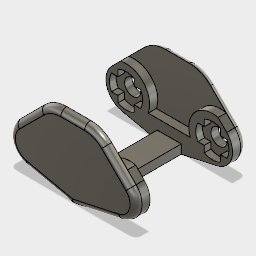
servo_bracket_shin (Autodesk Fusion 360 design; units mm, degrees)
Autodesk Fusion 360 part; units mm, degrees
sketch "スケッチ1" plane through (0, 0, 0) normal (0, 0, 1) x (1, 0, 0)
  line L0 (0, 0) -> (-4, 0)
  line L1 (0, 0) -> (4, 0)
  line L2 (-4, 0) -> (-15.8267, 2.557)
  line L3 (-4, 0) -> (8.1, 0) construction
  line L4 (4, 0) -> (15.8267, 2.557)
  line L5 (4, 0) -> (16.1, 0) construction
  line L6 (-15.8267, 2.557) -> (-14.4003, 9.1546)
  line L7 (15.8267, 2.557) -> (14.4003, 9.1546)
  circle A0 centre (14.4003, 9.1546) radius 6.75
  circle A1 centre (-14.4003, 9.1546) radius 6.75
  line L8 (14.4003, 9.1546) -> (15.8267, 2.557)
  line L9 (14.4003, 9.1546) -> (19.1733, 13.9276)
  line L10 (14.4003, 9.1546) -> (21.1503, 9.1546) construction
  line L11 (-14.4003, 9.1546) -> (-19.1733, 13.9276)
  line L12 (-14.4003, 9.1546) -> (-7.6503, 9.1546) construction
  line L13 (19.1733, 13.9276) -> (11.0592, 22.0416)
  line L14 (11.0592, 22.0416) -> (3.9881, 14.9705)
  line L15 (11.0592, 22.0416) -> (21.0592, 22.0416) construction
  line L16 (3.9881, 14.9705) -> (3.9881, 24.9705)
  arc A2 (11.0592, 22.0416) -> (3.9881, 24.9705) centre (3.9881, 14.9705) ccw
  line L17 (-19.1733, 13.9276) -> (-11.0592, 22.0416)
  line L18 (-11.0592, 22.0416) -> (-3.9881, 14.9705)
  line L19 (-3.9881, 14.9705) -> (-3.9881, 24.9705)
  line L20 (-3.9881, 24.9705) -> (3.9881, 24.9705)
  arc A3 (-3.9881, 24.9705) -> (-11.0592, 22.0416) centre (-3.9881, 14.9705) ccw
  circle A4 centre (-14.4003, 9.1546) radius 2.7
  circle A5 centre (14.4003, 9.1546) radius 2.7
  circle A6 centre (-14.4003, 9.1546) radius 2
  circle A7 centre (14.4003, 9.1546) radius 2
  circle A8 centre (-14.4003, 9.1546) radius 7.875
  circle A9 centre (14.4003, 9.1546) radius 7.875
  line L21 (0, 0) -> (0, 6.4) construction
  line L22 (0, 6.4) -> (-7.0228, 6.4)
  line L23 (0, 6.4) -> (7.0228, 6.4)
  line L24 (-4, 0) -> (4, 0)
  line L25 (4, 0) -> (4, 3)
  line L26 (4, 3) -> (-4, 3)
  line L27 (-4, 3) -> (-4, 0)
  dimension "d1" = 4
  dimension "d2" = 4
  dimension "d3" = 167.8
  dimension "d4" = 12.1
  dimension "d5" = 12.2
  dimension "d6" = 12.1
  dimension "d7" = 6.75
  dimension "d8" = 6.75
  dimension "d9" = 6.75
  dimension "d10" = 45
  dimension "d11" = 6.75
  dimension "d12" = 135
  dimension "d13" = 11.475
  dimension "d16" = 10
  dimension "d18" = 10
  dimension "d19" = 11.475
  dimension "d20" = 10
  dimension "d21" = 10
  dimension "d28" = 5.4
  dimension "d29" = 5.4
  dimension "d30" = 4
  dimension "d31" = 4
  dimension "d32" = 15.75
  dimension "d33" = 15.75
  dimension "d34" = 6.4
  dimension "d53" = 3
  constraint horizontal L3
  constraint horizontal L5
  constraint perpendicular L2 L6
  constraint perpendicular L4 L7
  constraint coincident A0
  constraint coincident A1
  constraint tangent L2 A1
  constraint horizontal L10
  constraint horizontal L12
  constraint perpendicular L9 L13
  constraint perpendicular L13 L14
  constraint horizontal L15
  constraint perpendicular L11 L17
  constraint tangent A2 L20
  constraint concentric A4 A6
  constraint concentric A5 A7
  constraint concentric A6 A8
  constraint concentric A7 A9
  constraint coincident A8
  constraint perpendicular L21 L22
  constraint coincident A9
  constraint perpendicular L21 L23
  constraint perpendicular L24 L25
  constraint parallel L24 L26
  constraint parallel L25 L27
  constraint parallel L5 L24
  measures "d3" angle of L2 L3
  measures "d5" angle of L4 L5
  measures "d10" angle of L9 L10
  measures "d12" angle of L11 L12
  measures "d28" diameter of A4
  measures "d29" diameter of A5
  measures "d30" diameter of A6
  measures "d31" diameter of A7
  measures "d32" diameter of A8
  measures "d33" diameter of A9
extrude "押し出し2" add sketch "スケッチ1" against normal blind 4.7 contours L0 L1 L24 L25 L26 L27 | L2 L4 A8 A9 L22 L23 L25 L26 L27 | L2 A1 L17 A8 | L4 A0 L13 A9 | L6 A1 L11 A4 | L6 A1 L11 A4 | L7 A0 L8 L9 A5 | L7 A0 L8 L9 A5 | L6 L11 A4 A6 | L6 L11 A4 A6 | L7 L8 L9 A5 A7 | L7 L8 L9 A5 A7 picked at (-7.6137, 5.9962) picked at (7.6206, 5.9818) makes body 1
extrude "押し出し3" add sketch "スケッチ1" against normal blind 2 contours L0 L1 L24 L25 L26 L27 | L2 L4 A8 A9 L22 L23 L25 L26 L27 | L2 A1 L17 A8 | L4 A0 L13 A9 | L6 A1 L11 A4 | L6 A1 L11 A4 | L13 L14 L16 L17 L18 L19 L20 A8 A9 L22 L23 | L7 A0 L8 L9 A5 | L7 A0 L8 L9 A5 | L6 L11 A4 A6 | L6 L11 A4 A6 | L18 L19 A3 | L7 L8 L9 A5 A7 | L7 L8 L9 A5 A7 | L6 L11 A6 | L6 L11 A6 | L7 L8 L9 A7 | L7 L8 L9 A7 | L14 L16 A2 picked at (-7.6137, 5.9962) picked at (7.6206, 5.9818) bodies 1
ref_plane "作業平面2" through (0, 15.6853, -18.45) normal (0, 0, 1) x (1, 0, 0)
mirror "ミラー4" about plane through (0, 15.6853, -18.45) normal (0, 0, 1) of bodies 1 makes body 2
sketch "スケッチ2" plane through (0, 0, -32.2) normal (0, 0, 1) x (1, 0, 0)
  circle A0 centre (-14.4003, 9.1546) radius 2
  circle A1 centre (14.4003, 9.1546) radius 2
  arc A2 (-7.0228, 6.4) -> (-16.3051, 16.7958) centre (-14.4003, 9.1546) ccw
  line L0 (-16.3051, 16.7958) -> (-19.1733, 13.9276)
  arc A3 (-19.1733, 13.9276) -> (-15.8267, 2.557) centre (-14.4003, 9.1546) ccw
  line L1 (-15.8267, 2.557) -> (-4, 0)
  line L2 (-4, 0) -> (4, 0)
  line L3 (4, 0) -> (15.8267, 2.557)
  arc A4 (15.8267, 2.557) -> (19.1733, 13.9276) centre (14.4003, 9.1546) ccw
  line L4 (19.1733, 13.9276) -> (16.3051, 16.7958)
  arc A5 (16.3051, 16.7958) -> (7.0228, 6.4) centre (14.4003, 9.1546) ccw
  line L5 (7.0228, 6.4) -> (-7.0228, 6.4)
  circle A6 centre (14.4003, 9.1546) radius 2.7
  circle A7 centre (-14.4003, 9.1546) radius 2.7
  circle A8 centre (14.4003, 9.1546) radius 5.55
  circle A9 centre (-14.4003, 9.1546) radius 5.55
  line L6 (17.1003, 6.4546) -> (11.7003, 6.4546)
  line L7 (11.7003, 6.4546) -> (11.7003, 11.8546)
  line L8 (11.7003, 11.8546) -> (17.1003, 11.8546)
  line L9 (17.1003, 11.8546) -> (17.1003, 6.4546)
  line L10 (17.1003, 6.4546) -> (11.7003, 11.8546) construction
  line L11 (11.7003, 6.4546) -> (17.1003, 11.8546) construction
  line L12 (-11.7003, 6.4546) -> (-17.1003, 6.4546)
  line L13 (-17.1003, 6.4546) -> (-17.1003, 11.8546)
  line L14 (-17.1003, 11.8546) -> (-11.7003, 11.8546)
  line L15 (-11.7003, 11.8546) -> (-11.7003, 6.4546)
  line L16 (-11.7003, 6.4546) -> (-17.1003, 11.8546) construction
  line L17 (-17.1003, 6.4546) -> (-11.7003, 11.8546) construction
  line L18 (-11.7003, 11.8546) -> (-11.7003, 14.0036)
  line L19 (-11.7003, 11.8546) -> (-9.5513, 11.8546)
  line L20 (-11.7003, 6.4546) -> (-9.5513, 6.4546)
  line L21 (-11.7003, 6.4546) -> (-11.7003, 4.3056)
  line L22 (-17.1003, 6.4546) -> (-17.1003, 4.3056)
  line L23 (-17.1003, 6.4546) -> (-19.2493, 6.4546)
  line L24 (-17.1003, 11.8546) -> (-19.2493, 11.8546)
  line L25 (-17.1003, 11.8546) -> (-17.1003, 14.0036)
  line L26 (17.1003, 11.8546) -> (19.2493, 11.8546)
  line L27 (17.1003, 11.8546) -> (17.1003, 14.0036)
  line L28 (11.7003, 11.8546) -> (11.7003, 14.0036)
  line L29 (11.7003, 11.8546) -> (9.5513, 11.8546)
  line L30 (11.7003, 6.4546) -> (9.5513, 6.4546)
  line L31 (11.7003, 6.4546) -> (11.7003, 4.3056)
  line L32 (17.1003, 6.4546) -> (17.1003, 4.3056)
  line L33 (17.1003, 6.4546) -> (19.2493, 6.4546)
  dimension "d41" = 5.4
  dimension "d42" = 5.4
  dimension "d43" = 11.1
  dimension "d44" = 11.1
  dimension "d45" = 5.4
  dimension "d46" = 5.4
  dimension "d47" = 5.4
  dimension "d48" = 5.4
  constraint concentric A1 A6
  constraint concentric A0 A7
  constraint concentric A6 A8
  constraint concentric A7 A9
  constraint perpendicular L6 L7
  constraint parallel L6 L8
  constraint parallel L7 L9
  constraint horizontal L6
  constraint coincident L10
  constraint coincident L11
  constraint perpendicular L12 L13
  constraint parallel L12 L14
  constraint parallel L13 L15
  constraint horizontal L12
  constraint coincident L16
  constraint coincident L17
  constraint coincident A9
  constraint perpendicular L14 L18
  constraint perpendicular L18 L19
  constraint perpendicular L15 L20
  constraint perpendicular L20 L21
  constraint perpendicular L12 L22
  constraint perpendicular L22 L23
  constraint perpendicular L13 L24
  constraint perpendicular L24 L25
  constraint coincident A8
  constraint perpendicular L25 L26
  constraint perpendicular L26 L27
  constraint perpendicular L8 L28
  constraint perpendicular L28 L29
  constraint perpendicular L7 L30
  constraint perpendicular L30 L31
  constraint perpendicular L6 L32
  constraint perpendicular L32 L33
  measures "d41" diameter of A6
  measures "d42" diameter of A7
  measures "d43" diameter of A8
  measures "d44" diameter of A9
extrude "押し出し4" cut sketch "スケッチ2" against normal blind 10 contours A0 | A1 | A6 | A7 bodies 2
extrude "押し出し5" cut sketch "スケッチ2" against normal blind 2.2 contours A0 | A1 | A6 | A6 L6 L9 | A6 L8 L9 | A8 L9 L26 L33 | A6 L7 L8 | A8 L8 L27 L28 | A6 L6 L7 | A8 L6 L31 L32 | A8 L7 L29 L30 | A7 | A7 L12 L15 | A7 L14 L15 | A9 L15 L19 L20 | A7 L13 L14 | A9 L14 L18 L25 | A7 L12 L13 | A9 L12 L21 L22 | A9 L13 L23 L24 bodies 2
extrude "押し出し6" add sketch "スケッチ1" against normal blind 33 contours L0 L1 L24 L25 L26 L27 bodies 1 2
fillet "フィレット1" radius 2 9 edges at (-9.9134, 1.2785, -36.9) (-20.8757, 7.2488, -36.9) (-15.1162, 17.9846, -36.9) (-7.815, 24.2093, -36.9) (0, 24.9705, -36.9) (7.815, 24.2093, -36.9) (15.1162, 17.9846, -36.9) (20.8757, 7.2488, -36.9) (9.9134, 1.2785, -36.9) on bodies 1
fillet "フィレット2" radius 2 9 edges at (9.9134, 1.2785, 0) (20.8757, 7.2488, 0) (15.1162, 17.9846, 0) (7.815, 24.2093, 0) (0, 24.9705, 0) (-7.815, 24.2093, 0) (-15.1162, 17.9846, 0) (-20.8757, 7.2488, 0) (-9.9134, 1.2785, 0) on bodies 1
equation "d39 = ( -36.9 / 2 ) * 1 mm"
